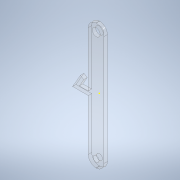
# Autodesk Inventor part: part_0.22 Lexan Intake Arm
Saved by Autodesk Inventor 2021.1 (Build 251245000, 245)
## iProperties
Created: 2021-02-24
Part Number: part_0.22 Lexan Intake Arm
Material: Generic
Document SubType Name: Modeling
Designer: JavDiazV
Density: 1 g/cm^3
Appearance: Polycarbonate - Clear
Author: JavDiazV
Autodesk Inventor part; units mm, degrees
ref_plane "YZ Plane" through (0, 0, 0) normal (1, 0, 0) x (0, 1, 0)
ref_plane "XZ Plane" through (0, 0, 0) normal (0, 1, 0) x (-1, 0, 0)
ref_plane "XY Plane" through (0, 0, 0) normal (0, 0, 1) x (1, 0, 0)
sketch "Sketch1" plane through (0, 0, 0) normal (0, 0, 1) x (1, 0, 0)
  point P0 (0, 0)
sketch "Sketch2" plane through (0, 0, 0) normal (0, 1, 0) x (-1, 0, 0)
  point P0 (0, 0)
sketch "Sketch3" plane through (0, 0, 0) normal (0, 0, 1) x (1, 0, 0)
  line L0 (13.1045, 101.3977) -> (-12.2955, 101.3977)
  line L1 (-12.2955, 101.3977) -> (-12.2955, -101.8023)
  line L2 (-12.2955, -101.8023) -> (13.1045, -101.8023)
  line L3 (13.1045, -101.8023) -> (13.1045, 101.3977)
  arc A0 (13.1045, 88.6986) -> (-12.2955, 88.6986) centre (0.4045, 88.6986) ccw
  line L4 (-12.2955, 88.6986) -> (13.1045, 88.6986) construction
  line L5 (-12.2955, 88.6986) -> (13.1045, 88.6986) construction
  arc A1 (-12.2955, -89.1032) -> (13.1045, -89.1032) centre (0.4045, -89.1032) ccw
  line L6 (-12.2955, -89.1032) -> (13.1045, -89.1032) construction
  line L7 (-12.2955, -89.1032) -> (13.1045, -89.1032) construction
  circle A2 centre (0.4045, -89.1032) radius 4.7625
  line L8 (13.1045, -25.5967) -> (114.815, -25.5967) construction
  point P0 (0, 0)
  point P1 (0.2548, -101.8023)
  point P2 (0.5541, -101.8023)
  point P3 (0.5519, 101.3977)
  point P4 (0.257, 101.3977)
  dimension "d0" = 25.4
  dimension "d1" = 203.2
  dimension "d2" = 360
  dimension "d3" = 360
  dimension "d4" = 9.525
  constraints: 18 end point, 5 point on line, 4 horizontal, 4 point on circle, 4 tangent, 3 centre point, 2 collinear, 2 parallel, 1 coincident, 1 perpendicular
  measures "d0" distance of L2.end L1.end
  measures "d1" distance of L1.end L0.end
  measures "d4" diameter of A2
extrude "Extrusion1" add sketch "Sketch3" along normal blind 5.588 contours A0 L3 A1 L1
sketch "Sketch4" plane through (0, 0, 5.588) normal (0, 0, 1) x (1, 0, 0)
  circle A0 centre (0.4045, 88.6968) radius 4.7625
  line L0 (-12.2955, 88.6986) -> (-12.2955, -89.1032) projected
  arc A1 (-12.2955, -89.1032) -> (0.2548, -101.8023) centre (0.4045, -89.1032) ccw projected
  point P0 (0, 0)
  dimension "d12" = 9.525
  dimension "d13" = 12.7
  dimension "d14" = 177.8
  constraints: 1 centre point
  measures "d12" diameter of A0
  measures "d13" distance from line of L0 A0.centre
  measures "d14" distance of A1.centre A0.centre
extrude "Extrusion2" cut sketch "Sketch4" against normal through all
sketch "Sketch5" plane through (0, 0, 5.588) normal (0, 0, 1) x (1, 0, 0)
  line L0 (-12.2955, 88.6986) -> (-12.2955, -89.1032) projected
  line L1 (-12.2955, -0.2023) -> (-12.2955, 6.1477)
  line L2 (-12.2955, -0.2023) -> (-12.2955, -6.5523)
  line L3 (-12.2955, -6.5523) -> (-37.6955, -6.5523)
  line L4 (-37.6955, -6.5523) -> (-24.9955, 15.4447)
  line L5 (-24.9955, 15.4447) -> (-19.4963, 12.2697)
  line L6 (-19.4963, 12.2697) -> (-26.697, -0.2023)
  line L7 (-26.697, -0.2023) -> (-12.2955, -0.2023)
  point P0 (0, 0)
  dimension "d24" = 25.4
  dimension "d25" = 25.4
  dimension "d26" = 60
  dimension "d27" = 6.35
  constraints: 14 end point, 2 perpendicular, 2 point on line, 1 horizontal, 1 midpoint, 1 parallel
  measures "d24" distance of L2.end L3.end
  measures "d25" distance of L3.end L4.end
  measures "d26" angle of L3 L4
  measures "d27" distance of L4.end L5.end
extrude "Extrusion3" add sketch "Sketch5" against normal blind 5.588
sketch "Sketch6" plane through (0, 0, 5.588) normal (0, 0, 1) x (1, 0, 0)
  arc A0 (13.1045, 88.6986) -> (0.5519, 101.3977) centre (0.4045, 88.6986) ccw projected
  line L0 (0.5519, 101.3977) -> (0.4045, 88.6986)
  circle A1 centre (0.5519, 88.6986) radius 6.35
  point P0 (0, 0)
  dimension "d30" = 12.7
  constraints: 2 end point, 1 centre point, 1 point on circle
  measures "d30" diameter of A1
extrude "Extrusion4" cut sketch "Sketch6" against normal through all
body "Solid1"
